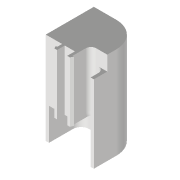
# Autodesk Inventor part: Corner1
Saved by Autodesk Inventor 2021 (Build 250183000, 183)
## iProperties
Created: 2021-07-29
Part Number: Corner1
Material: Generisch
Document SubType Name: Modeling
Designer: Rama
Density: 1 g/cm^3
Appearance: Vorgabe
Author: Rama
Autodesk Inventor part; units mm, degrees
ref_plane "YZ Plane" through (0, 0, 0) normal (1, 0, 0) x (0, 1, 0)
ref_plane "XZ Plane" through (0, 0, 0) normal (0, 1, 0) x (-1, 0, 0)
ref_plane "XY Plane" through (0, 0, 0) normal (0, 0, 1) x (1, 0, 0)
sketch "Skizze1" plane through (0, 0, 0) normal (0, 1, 0) x (-1, 0, 0)
  line L0 (10, 10) -> (-10, 10)
  line L1 (-10, 10) -> (-10, -10)
  line L2 (-10, -10) -> (10, -10)
  line L3 (10, -10) -> (10, 10)
  line L4 (10, 10) -> (-10, -10) construction
  line L5 (-10, 10) -> (10, -10) construction
  point P0 (0, 0)
  dimension "d0" = 20
  dimension "d1" = 20
  constraints: 12 end point, 2 midpoint, 2 parallel, 1 horizontal, 1 perpendicular
  measures "d0" distance of L2.end L1.end
  measures "d1" distance of L1.end L0.end
extrude "Extrusion1" add sketch "Skizze1" along normal blind 34.5
sketch "Skizze2" plane through (0, 0, 0) normal (0, -1, 0) x (1, 0, 0)
  line L0 (-8.9654, -8) -> (-1.6431, -8)
  line L1 (8, 1.6431) -> (8, 9.2)
  line L2 (-10, 10) -> (10, 10)
  line L3 (-10, -10) -> (-10, 10)
  line L4 (8, 10) -> (-10, 10)
  line L5 (-10, 10) -> (-10, -8)
  line L6 (-10, -8) -> (8, -8)
  line L7 (8, -8) -> (8, 10)
  line L8 (10, 10) -> (10, -10)
  line L9 (-10, 10) -> (10, 10)
  line L10 (-10, -10) -> (-10, 10)
  line L11 (10, -10) -> (-10, -10)
  circle A0 centre (-1.6431, 1.6431) radius 9.6431
  point P0 (0, 0)
  constraints: 24 end point, 2 point on line, 3 other
extrude "Extrusion2" cut sketch "Skizze2" against normal through all contours L0 L6 L7 L1 L2 L8 L11 L3 | A0 L7 L6
sketch "Skizze3" plane through (0, 34.5, 0) normal (0, 1, 0) x (1, 0, 0)
  line L0 (0.9, -9.6) -> (0.9, -12.8936) projected
  line L1 (0.9, -12.8936) -> (1.9, -12.8936) projected
  line L2 (1.9, -12.8936) -> (2.4, -11.85) projected
  line L3 (2.4, -11.85) -> (1.9, -11.85) projected
  line L4 (1.9, -12.8936) -> (1.9, -9.6) projected
  line L5 (-2.9, -12.8936) -> (-2.9, -9.6) projected
  line L6 (-3.9, -9.6) -> (-3.9, -12.8936) projected
  line L7 (-3.9, -11.85) -> (-4.4, -11.85) projected
  line L8 (-4.4, -11.85) -> (-3.9, -12.8936) projected
  line L9 (-3.9, -12.8936) -> (-2.9, -12.8936) projected
  line L10 (0.9, -12.8936) -> (1.9, -12.8936)
  line L11 (1.9, -12.8936) -> (1.9, -9.6)
  line L12 (1.9, -9.6) -> (0.9, -9.6)
  line L13 (0.9, -9.6) -> (0.9, -12.8936)
  line L14 (-2.9, -12.8936) -> (-3.9, -12.8936)
  line L15 (-3.9, -12.8936) -> (-3.9, -9.6)
  line L16 (-3.9, -9.6) -> (-2.9, -9.6)
  line L17 (-2.9, -9.6) -> (-2.9, -12.8936)
  point P0 (0, 0)
  constraints: 16 end point, 4 parallel, 2 horizontal, 2 perpendicular
extrude "Extrusion3" add sketch "Skizze3" against normal up to surface (34.5 mm away)
sketch "Skizze4" plane through (0, 0, 0) normal (0, -1, 0) x (1, 0, 0)
  line L0 (-8.9657, 0.9754) -> (-0.9754, 8.9657) projected
  line L1 (-0.9754, 8.9657) -> (0.1723, 7.818) projected
  line L2 (-0.4527, 5.1738) -> (0.1723, 7.818) projected
  line L3 (-0.7807, 3.7863) -> (-3.7863, 0.7807) projected
  line L4 (-5.174, 0.4527) -> (-7.818, -0.1723) projected
  line L5 (-7.818, -0.1723) -> (-8.9657, 0.9754) projected
  line L6 (-10, 10) -> (-3.9, 10) projected
  line L7 (-8.8, 10) -> (2, 10)
  line L8 (2, 10) -> (2, 3)
  line L9 (-3, -2) -> (-5.8, -2)
  line L10 (-8.8, -2) -> (-8.8, 10)
  line L11 (-10, -8) -> (-10, 10) projected
  line L12 (-8.8, 10) -> (-10, 10)
  line L13 (-10, 10) -> (-10, -2)
  line L14 (-10, -2) -> (-8.8, -2)
  line L15 (-8.8, 1) -> (-8.8, 10)
  arc A0 (-3, -2) -> (2, 3) centre (-3, 3) ccw
  arc A1 (-8.8, 1) -> (-5.8, -2) centre (-5.8, 1) ccw
  line L16 (-8.8, 10) -> (4, 10)
  line L17 (4, 10) -> (4, 19)
  line L18 (4, 19) -> (-8.8, 19)
  line L19 (-8.8, 19) -> (-8.8, 10)
  point P0 (0, 0)
  point P1 (2, -2)
  point P2 (2, 10)
  dimension "d8" = 12
  dimension "d9" = 1.2
  dimension "d10" = 5
  dimension "d11" = 3
  constraints: 24 end point, 6 parallel, 6 point on line, 4 point on circle, 4 tangent, 3 horizontal, 3 perpendicular, 2 centre point
  measures "d8" distance of L7.end point (2, -2)
  measures "d9" distance of L13.end L14.end
  measures "d10" radius of A0
  measures "d11" radius of A1
extrude "Extrusion4" cut sketch "Skizze4" against normal blind 12 contours L10 L6 L7 L8 A0 L9 A1 | L19 L18 L17 L16 L7 L6
sketch "Skizze5" plane through (8, 0, 10) normal (0, 0, 1) x (1, 0, 0)
  line L0 (-6.1, 34.5) -> (0, 34.5) projected
  line L1 (0, 34.5) -> (-6.1, 34.5)
  line L2 (-6.1, 34.5) -> (-6.1, 29)
  line L3 (-6.1, 29) -> (0, 29)
  line L4 (0, 29) -> (0, 34.5)
  line L5 (0, 29) -> (-1.2, 29)
  line L6 (-1.2, 29) -> (-1.2, 0)
  line L7 (-1.2, 0) -> (0, 0)
  line L8 (0, 0) -> (0, 29)
  line L9 (-6, 0) -> (0, 0) projected
  line L10 (-1.2, 29) -> (-6.1, 29)
  line L11 (-6.1, 29) -> (-6.1, 0)
  line L12 (-6.1, 0) -> (-1.2, 0)
  line L13 (-1.2, 0) -> (-1.2, 29)
  point P0 (-8, 0)
  dimension "d14" = 6.1
  dimension "d15" = 1.2
  dimension "d16" = 4.9
  constraints: 24 end point, 6 parallel, 3 horizontal, 3 perpendicular, 1 point on line
  measures "d14" distance of L3.end L2.end
  measures "d15" distance of L7.end L6.end
  measures "d16" distance of L12.end L11.end
extrude "Extrusion5" cut sketch "Skizze5" against normal blind 5 contours L0 L4 L3 L2 | L3 L6 L9 L12 L11
fillet "Rundung1" radius 2 1 edges at (6.8, 14.5, 5)
fillet "Rundung2" radius 4 1 edges at (2, 6, 5)
fillet "Rundung3" radius 2 2 edges at (4.9661, 12, 5.0069) (3.35, 12, 5)
fillet "Rundung4" radius 2 3 edges at (1.9, 12.5858, 4.4142) (1.9, 21.5, 5) (1.9, 31.75, 5)
